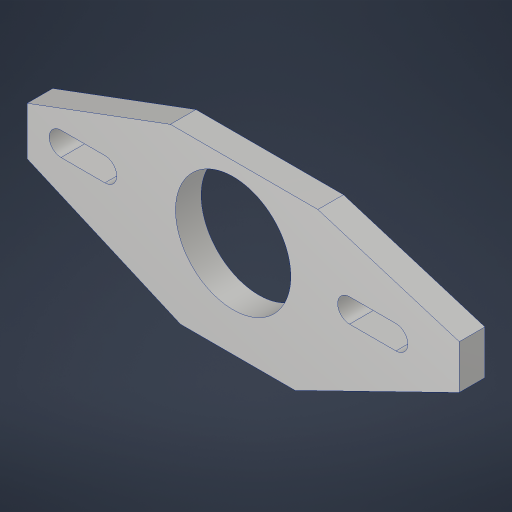
# Autodesk Inventor part: EL2-CGB-010
Saved by Autodesk Inventor 2023.4 (Build 274418000, 418)
## iProperties
Created: 2025-01-24
Part Number: EL2-CGB-010
Material: Aluminum 6061
Document SubType Name: Modeling
Designer: brand
Density: 2.7 g/cm^3
Appearance: Aluminum - Flat
Author: brand
Autodesk Inventor part; units mm, degrees
ref_plane "YZ Plane" through (0, 0, 0) normal (1, 0, 0) x (0, 1, 0)
ref_plane "XZ Plane" through (0, 0, 0) normal (0, 1, 0) x (-1, 0, 0)
ref_plane "XY Plane" through (0, 0, 0) normal (0, 0, 1) x (1, 0, 0)
sketch "Sketch1" plane through (0, 0, 0) normal (0, 0, 1) x (1, 0, 0)
  circle A0 centre (0, 0) radius 14.2875
  line L0 (-42.6642, 0) -> (-31.7972, 0) construction
  line L1 (-42.6642, -2.9337) -> (-31.7972, -2.9337)
  line L2 (-31.7972, 2.9337) -> (-42.6642, 2.9337)
  arc A1 (-42.6642, 2.9337) -> (-42.6642, -2.9337) centre (-42.6642, 0) ccw
  arc A2 (-31.7972, -2.9337) -> (-31.7972, 2.9337) centre (-31.7972, 0) ccw
  line L3 (28.8375, 0) -> (40.3345, 0) construction
  line L4 (28.8375, -2.9431) -> (40.3345, -2.9431)
  line L5 (40.3345, 2.9431) -> (28.8375, 2.9431)
  arc A3 (28.8375, 2.9431) -> (28.8375, -2.9431) centre (28.8375, 0) ccw
  arc A4 (40.3345, -2.9431) -> (40.3345, 2.9431) centre (40.3345, 0) ccw
  line L6 (-15.5732, 17.7397) -> (-51.0822, 4.5132)
  line L7 (-51.0822, 4.5132) -> (-51.0822, -7.4026)
  line L8 (-51.0822, -7.4026) -> (-13.0709, -23.9059)
  line L9 (-13.0709, -23.9059) -> (15.3482, -23.9059)
  line L10 (15.3482, -23.9059) -> (56.0406, -4.0066)
  line L11 (56.0406, -4.0066) -> (56.0406, 6.8964)
  line L12 (56.0406, 6.8964) -> (20.9914, 17.7397)
  line L13 (20.9914, 17.7397) -> (-15.5732, 17.7397)
  point P0 (-37.2307, 0)
  point P1 (34.586, 0)
  dimension "d0" = 28.575
  constraints: 32 end point, 8 point on circle, 8 tangent, 5 centre point, 3 perpendicular, 2 midpoint, 2 parallel, 2 point on line, 1 coincident, 1 horizontal, 1 vertical
  measures "d0" diameter of A0
extrude "Extrusion1" add sketch "Sketch1" along normal blind 6.35
body "Solid1"
